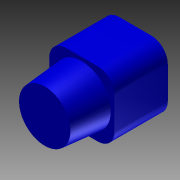
# Autodesk Inventor part: rangefinder model
Saved by Autodesk Inventor 2012 (Build 160160000, 160)
## iProperties
Created: 2011-10-07
Part Number: rangefinder model
Material: Default
Document SubType Name: Modeling
Designer: Antonella
Density: 1 g/cm^3
Author: Antonella
Autodesk Inventor part; units mm, degrees
ref_plane "YZ Plane" through (0, 0, 0) normal (1, 0, 0) x (0, 1, 0)
ref_plane "XZ Plane" through (0, 0, 0) normal (0, 1, 0) x (-1, 0, 0)
ref_plane "XY Plane" through (0, 0, 0) normal (0, 0, 1) x (1, 0, 0)
sketch "Sketch1" plane through (0, 0, 0) normal (0, 0, 1) x (1, 0, 0)
  line L0 (-35, 0) -> (35, 0) projected
  line L1 (0, -35) -> (0, 35) projected
  line L2 (-25, 25) -> (25, 25)
  line L3 (25, 25) -> (25, -25)
  line L4 (25, -25) -> (-25, -25)
  line L5 (-25, -25) -> (-25, 25)
  point P0 (0, 0)
  point P1 (-25, 0)
  point P2 (0, 25)
  dimension "d0" = 50
  constraints: 8 end point, 2 midpoint, 2 parallel, 2 perpendicular, 1 horizontal, 1 horizontal alignment, 1 vertical alignment
  measures "d0" distance of L4.end L2.start
extrude "Extrusion1" add sketch "Sketch1" along normal blind 41
sketch "Sketch2" plane through (0, 0, 41) normal (0, 0, 1) x (1, 0, 0)
  circle A0 centre (0, 0) radius 22.225
  dimension "d3" = 44.45
  constraints: 1 centre point, 1 coincident
  measures "d3" diameter of A0
extrude "Extrusion2" add sketch "Sketch2" along normal blind 28.5 draft -5
fillet "Fillet1" radius 12.7 4 edges at (25, 25, 20.5) (25, -25, 20.5) (-25, 25, 20.5) (-25, -25, 20.5)
body "Solid1"
